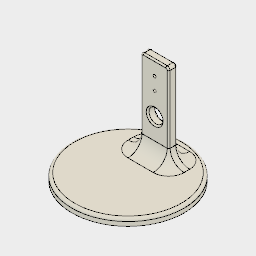
WebCam_Stand_v9 (Autodesk Fusion 360 design; units mm, degrees)
Autodesk Fusion 360 part; units mm, degrees
sketch "Sketch1" plane through (0, 0, 0) normal (0, 1, 0) x (1, 0, 0)
  circle A0 centre (0, 0) radius 80
  dimension "d1" = 160
  measures "d1" diameter of A0
extrude "Extrude1" add sketch "Sketch1" along normal blind 10 makes body 1
fillet "Fillet1" radius 4 1 edges at (-74.5862, 10, 28.9292) on bodies 1
sketch "Sketch2" plane through (0, 0, 0) normal (0, 1, 0) x (1, 0, 0)
  line L0 (125, 0) -> (165, 0)
  line L1 (165, 0) -> (165, 120)
  line L2 (165, 120) -> (125, 120)
  line L3 (125, 120) -> (125, 0)
  circle A0 centre (145, 100) radius 2
  circle A1 centre (145, 81.9961) radius 2
  circle A2 centre (145, 50) radius 10
  point P0 (145, 100)
  dimension "d5" = 120
  dimension "d6" = 40
  dimension "d7" = 4
  dimension "d8" = 4
  dimension "d9" = 20
  measures "d5" distance of L0.start L2.end
  measures "d6" distance of L0.start L0.end
  measures "d7" diameter of A0
  measures "d8" diameter of A1
  measures "d9" diameter of A2
extrude "Extrude2" add sketch "Sketch2" along normal blind 12 separate body makes body 2
sketch "Sketch3" plane through (0, 0, 0) normal (0, 1, 0) x (1, 0, 0)
  line L0 (145, 104) -> (141.5359, 102)
  line L1 (141.5359, 102) -> (141.5359, 98)
  line L2 (141.5359, 98) -> (145, 96)
  line L3 (145, 96) -> (148.4641, 98)
  line L4 (148.4641, 98) -> (148.4641, 102)
  line L5 (148.4641, 102) -> (145, 104)
  line L6 (145, 86) -> (141.5359, 84)
  line L7 (141.5359, 84) -> (141.5359, 80)
  line L8 (141.5359, 80) -> (145, 78)
  line L9 (145, 78) -> (148.4641, 80)
  line L10 (148.4641, 80) -> (148.4641, 84)
  line L11 (148.4641, 84) -> (145, 86)
  point P0 (145, 100)
  point P1 (145, 82)
extrude "Extrude3" cut sketch "Sketch3" along normal blind 4 contours L6 L7 L8 L9 L10 L11 bodies 2
sketch "Sketch4" plane through (0, 0, 0) normal (0, 1, 0) x (1, 0, 0)
  line L0 (145, 104) -> (141.5359, 102)
  line L1 (141.5359, 102) -> (141.5359, 98)
  line L2 (141.5359, 98) -> (145, 96)
  line L3 (145, 96) -> (148.4641, 98)
  line L4 (148.4641, 98) -> (148.4641, 102)
  line L5 (148.4641, 102) -> (145, 104)
  point P0 (145, 100)
extrude "Extrude4" cut sketch "Sketch4" along normal blind 4 bodies 2
fillet "Fillet2" radius 4 1 edges at (165, 6, -120) on bodies 2
fillet "Fillet3" radius 4 1 edges at (125, 6, -120) on bodies 2
fillet "Fillet4" radius 2 1 edges at (135.6767, 12, -53.6162) on bodies 2
fillet "Fillet5" radius 2 1 edges at (135.6767, 0, -53.6162) on bodies 2
move_body "Move1" bodies 2 to x (1, 0, 0) y (0, 0, 1) z (0, -1, 0) at (0, 0, 0)
move_body "Move2" bodies 2 to x (1, 0, 0) y (0, 1, 0) z (0, 0, 1) at (0, 10, 0)
move_body "Move3" bodies 2 to x (1, 0, 0) y (0, 1, 0) z (0, 0, 1) at (-145, 0, 0)
move_body "Move4" bodies 2 to x (1, 0, 0) y (0, 1, 0) z (0, 0, 1) at (0, 0, -50)
combine "Combine1" operation add target body 1 tool bodies 2
fillet "Fillet6" radius 2 5 edges at (20, 68, -50) (18.8284, 128.8284, -50) (0, 130, -50) (-18.8284, 128.8284, -50) (-20, 68, -50) on bodies 1
fillet "Fillet7" radius 2 5 edges at (20, 68, -38) (18.8284, 128.8284, -38) (0, 130, -38) (-18.8284, 128.8284, -38) (-20, 68, -38) on bodies 1
fillet "Fillet8" radius 20 8 edges at (-19.4142, 10, -38.5858) (-20, 10, -44) (-19.4142, 10, -49.4142) (0, 10, -50) (19.4142, 10, -49.4142) (20, 10, -44) (19.4142, 10, -38.5858) (0, 10, -38) on bodies 1
named bodies: "Webcam Stand", "Mounting Plate"
